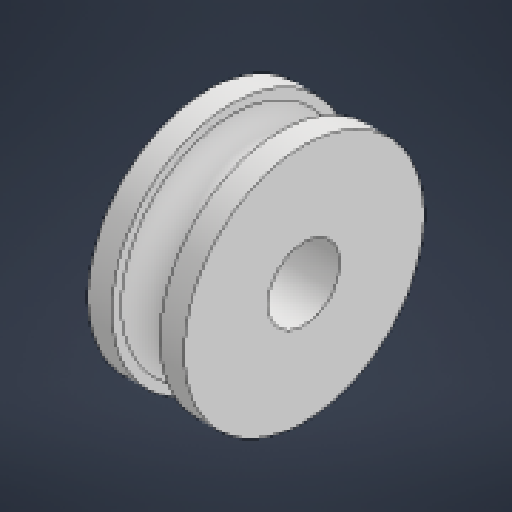
# Autodesk Inventor part: Pulley_Small
Saved by Autodesk Inventor 2024.2 (Build 282272000, 272)
## iProperties
Created: 2024-01-10
Part Number: Pulley_Small
Material: 一般
Document SubType Name: Modeling
Designer: Hanaoka
Density: 1 g/cm^3
Appearance: 既定
Author: Hanaoka
Autodesk Inventor part; units mm, degrees
ref_plane "YZ Plane" through (0, 0, 0) normal (1, 0, 0) x (0, 1, 0)
ref_plane "XZ Plane" through (0, 0, 0) normal (0, 1, 0) x (-1, 0, 0)
ref_plane "XY Plane" through (0, 0, 0) normal (0, 0, 1) x (1, 0, 0)
sketch "スケッチ1" plane through (0, 0, 0) normal (0, 0, 1) x (1, 0, 0)
  line L0 (-1, 0.75) -> (-1, 2.5)
  line L1 (1, 2.5) -> (1, 0.75)
  line L2 (-1, 0.75) -> (1, 0.75)
  line L3 (-1, 2.5) -> (-0.5, 2.5)
  line L4 (1, 2.5) -> (0.5, 2.5)
  line L5 (-0.5, 2.5) -> (-0.5, 2.3)
  line L6 (0.5, 2.5) -> (0.5, 2.3)
  arc A0 (-0.5, 2.3) -> (0.5, 2.3) centre (0, 2.3) ccw
  line L7 (0, 2.3) -> (0, 0.75) construction
  line L8 (-1.4, 0) -> (1.4, 0) projected
  point P0 (0, 0)
  dimension "d0" = 0.75
  dimension "d1" = 2
  dimension "d3" = 0.5
  dimension "d4" = 0.2
  dimension "d5" = 2.5
  constraints: 17 end point, 3 equal length, 3 vertical, 2 horizontal, 2 point on circle, 2 point on line, 1 centre point, 1 midpoint, 1 parallel, 1 tangent
  measures "d0" distance from line of point (0, 0) L2
  measures "d1" distance of L0.start L1.end
  measures "d3" distance of L1.start L4.end
  measures "d4" distance of L4.end L6.end
  measures "d5" distance from line of point (0, 0) L3
revolve "回転1" add sketch "スケッチ1" angle 360 about axis through (-10, 0, 0) along (1, 0, 0)
